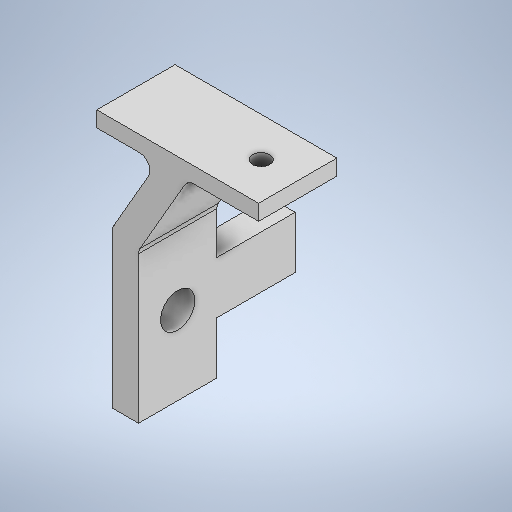
# Autodesk Inventor part: IR_senzor_hold_v2
Saved by Autodesk Inventor 2025 (Build 290162000, 162)
## iProperties
Created: 2025-02-23
Part Number: IR_senzor_hold_v2
Material: Všeobecné
Document SubType Name: Modeling
Designer: lukas
Density: 1 g/cm^3
Appearance: Výchozí
Author: lukas
## iProperties of the stored document IR_senzor_hold_v2_3D tisk.ipt
Created: 2025-02-23
Part Number: IR_senzor_hold_v2_3D tisk
Material: Všeobecné
Document SubType Name: Modeling
Designer: lukas
Density: 1 g/cm^3
Appearance: Výchozí
Author: lukas
Autodesk Inventor part; units mm, degrees
ref_plane "YZ Plane" through (0, 0, 0) normal (1, 0, 0) x (0, 1, 0)
ref_plane "XZ Plane" through (0, 0, 0) normal (0, 1, 0) x (-1, 0, 0)
ref_plane "XY Plane" through (0, 0, 0) normal (0, 0, 1) x (1, 0, 0)
sketch "Náčrt1" plane through (0, 0, 0) normal (0, 0, 1) x (1, 0, 0)
  line L0 (0, 33.6) -> (0, -33.6) projected
  line L1 (-11.7, 0) -> (31.7, 0) projected
  line L2 (-2.5, -24) -> (2.5, -24)
  line L3 (2.5, -24) -> (2.5, 4.6603)
  line L4 (2.5, 4.6603) -> (11.9338, 21)
  line L5 (11.9338, 21) -> (25.5, 21)
  line L6 (25.5, 21) -> (25.5, 24)
  line L7 (25.5, 24) -> (-5.5, 24)
  line L8 (-5.5, 24) -> (-5.5, 21)
  line L9 (-5.5, 21) -> (11.9338, 21)
  line L10 (-2.5, -24) -> (-2.5, 6)
  line L11 (-2.5, 6) -> (6.1603, 21)
  point P0 (0, 0)
  dimension "d0" = 5
  dimension "d2" = 5
  dimension "d3" = 30
  dimension "d4" = 15
  dimension "d5" = 31
  dimension "d6" = 3
  dimension "d7" = 60
  dimension "d8" = 3
  constraints: 20 end point, 4 perpendicular, 2 parallel, 2 point on line, 1 collinear, 1 horizontal, 1 vertical, 2 other
  measures "d0" distance between parallel lines of L10 L3
  measures "d2" distance between parallel lines of L11 L4
  measures "d3" distance of L2.start L10.end
  measures "d4" distance from line of L9 L10.end
  measures "d5" distance of L6.end L7.end
  measures "d6" distance between parallel lines of L5 L7
  measures "d7" angle of L9 L11
  measures "d8" distance between parallel lines of L10 L8
extrude "Vysunutí1" add sketch "Náčrt1" along normal blind 15 contours L7 L6 L5 L9 L0 | L0 L9 L8 L7 | L11 L9 L4 L3 L1 L0 | L0 L1 L10 L11 | L1 L3 L2 L0 | L0 L2 L10 L1
sketch "Náčrt2" plane through (-2.5, -24, 0) normal (-1, 0, 0) x (0, 0, 1)
  line L0 (0, 30) -> (0, 0) projected
  line L1 (0, 0) -> (15, 0) projected
  line L2 (15, 30) -> (15, 0) projected
  line L3 (0, 30) -> (15, 30) projected
  line L4 (0, -9.6) -> (0, 57.6) projected
  line L5 (-3, 24) -> (18, 24) projected
  point P0 (0, 24)
  point P1 (7.5, 15)
  dimension "d11" = 15
  dimension "d12" = 7.5
  measures "d11" distance from line of L3 point (7.5, 15)
  measures "d12" distance from line of L2 point (7.5, 15)
hole "Díra1" at (-2.5, -9, 7.5) direction (1, 0, 0) diameter 6.6 end through all clearance for "Šroub se šestihrannou hlavou ISO 24017" size "M6" standard "ISO"
sketch "Náčrt3" plane through (-5.5, 24, 0) normal (0, 1, 0) x (1, 0, 0)
  line L0 (31, 0) -> (0, 0) projected
  line L1 (0, 0) -> (0, -15) projected
  line L2 (31, -15) -> (0, -15) projected
  line L3 (31, 0) -> (31, -15) projected
  line L4 (5.5, 3) -> (5.5, -18) projected
  line L5 (37.2, 0) -> (-6.2, 0) projected
  point P0 (5.5, 0)
  point P1 (24, -7.5)
  point P2 (31, -7.5)
  dimension "d20" = 7.5
  dimension "d21" = 7
  constraints: 1 midpoint
  measures "d20" distance from line of L0 point (24, -7.5)
  measures "d21" distance of point (31, -7.5) point (24, -7.5)
hole "Díra2" at (18.5, 24, 7.5) direction (0, -1, 0) diameter 3.3 end through all
fillet "Zaoblení1" radius 2 4 edges at (11.9338, 21, 7.5) (6.1603, 21, 7.5) (2.5, 4.6603, 7.5) (-2.5, 6, 7.5)
sketch "Náčrt4" plane through (0, 0, 0) normal (0, 0, -1) x (-1, 0, 0)
  arc A0 (2.5, 5.4641) -> (2.2321, 6.4641) centre (0.5, 5.4641) ccw projected
  line L0 (-4.4282, 18) -> (2.2321, 6.4641) projected
  arc A1 (-2.6962, 21) -> (-4.4282, 18) centre (-2.6962, 19) ccw projected
  line L1 (5.5, 21) -> (-2.6962, 21) projected
  line L2 (5.5, 24) -> (5.5, 21) projected
  line L3 (-25.5, 24) -> (5.5, 24) projected
  line L4 (-25.5, 21) -> (-25.5, 24) projected
  line L5 (-13.0885, 21) -> (-25.5, 21) projected
  arc A2 (-11.3564, 20) -> (-13.0885, 21) centre (-13.0885, 19) ccw projected
  line L6 (-2.7679, 5.1244) -> (-11.3564, 20) projected
  arc A3 (-2.5, 4.1244) -> (-2.7679, 5.1244) centre (-4.5, 4.1244) ccw projected
  line L7 (-2.5, -24) -> (-2.5, 4.1244) projected
  line L8 (2.5, -24) -> (-2.5, -24) projected
  line L9 (2.5, 5.4641) -> (2.5, -24) projected
  line L10 (2.5, -14) -> (-2.5, -14)
  line L11 (-2.5, -14) -> (-2.5, -4)
  line L12 (-2.5, -4) -> (2.5, -4)
  line L13 (2.5, -4) -> (2.5, -14)
  point P0 (0, 0)
  dimension "d30" = 10
  dimension "d31" = 10
  constraints: 8 end point, 2 parallel, 2 point on line, 1 horizontal, 1 perpendicular
  measures "d30" distance of L12.end L10.start
  measures "d31" distance between parallel lines of L8 L10
extrude "Vysunutí2" add sketch "Náčrt4" along normal blind 15 contours L9 L10 L7 L12
